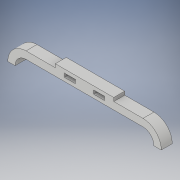
# Autodesk Inventor part: RadioPanelMountB
Saved by Autodesk Inventor 2018 (Build 220112000, 112)
## iProperties
Created: 2017-09-08
Part Number: RadioPanelMountB
Material: Generic
Document SubType Name: Modeling
Designer: Srinity
Density: 1 g/cm^3
Appearance: Default
Author: Srinity
Autodesk Inventor part; units mm, degrees
ref_plane "YZ Plane" through (0, 0, 0) normal (1, 0, 0) x (0, 1, 0)
ref_plane "XZ Plane" through (0, 0, 0) normal (0, 1, 0) x (-1, 0, 0)
ref_plane "XY Plane" through (0, 0, 0) normal (0, 0, 1) x (1, 0, 0)
sketch "Sketch1" plane through (0, 0, 0) normal (0, 0, 1) x (1, 0, 0)
  line L0 (-25.4, 9.398) -> (25.4, 9.398)
  line L1 (25.4, 9.398) -> (25.4, 6.35)
  line L2 (-25.4, 6.35) -> (-25.4, 9.398)
  line L3 (-50.8, 6.35) -> (-25.4, 6.35)
  line L4 (50.8, 6.35) -> (50.8, 0) construction
  line L5 (50.8, 0) -> (-50.8, 0)
  line L6 (-50.8, 0) -> (-50.8, 6.35) construction
  arc A0 (-50.8, 6.35) -> (-66.675, -9.525) centre (-50.8, -9.525) ccw
  arc A1 (38.1, 0) -> (66.675, -9.525) centre (50.8, -9.525) ccw construction
  arc A2 (-60.325, -9.525) -> (-50.8, -19.05) centre (-50.8, -9.525) ccw construction
  arc A3 (50.8, 0) -> (60.325, -9.525) centre (50.8, -9.525) ccw construction
  line L7 (25.4, 6.35) -> (50.8, 6.35)
  line L8 (-60.325, -9.525) -> (-66.675, -9.525)
  arc A4 (-50.8, 0) -> (-60.325, -9.525) centre (-50.8, -9.525) ccw
  arc A5 (60.325, -9.525) -> (50.8, 0) centre (50.8, -9.525) ccw
  arc A6 (-38.1, 0) -> (-50.8, 6.35) centre (-50.8, -9.525) ccw construction
  arc A7 (50.8, 6.35) -> (38.1, 0) centre (50.8, -9.525) ccw construction
  arc A8 (66.675, -9.525) -> (50.8, 6.35) centre (50.8, -9.525) ccw
  arc A9 (-66.675, -9.525) -> (-38.1, 0) centre (-50.8, -9.525) ccw construction
  arc A10 (-50.8, -19.05) -> (-50.8, 0) centre (-50.8, -9.525) ccw construction
  line L9 (66.675, -9.525) -> (60.325, -9.525)
  point P0 (0, 0)
  point P1 (50.8, 3.175)
  point P2 (-50.8, 3.175)
  dimension "d0" = 50.8
  dimension "d1" = 3.048
  dimension "d2" = 6.35
  dimension "d3" = 25.4
  dimension "d4" = 25.4
  dimension "d5" = 25.4
  dimension "d8" = 9.525
  constraints: 22 point on circle, 20 end point, 11 centre point, 6 tangent, 4 horizontal, 4 parallel, 4 point on line, 3 midpoint, 3 perpendicular, 2 coincident, 2 collinear, 2 equal radius, 2 vertical alignment
  measures "d0" distance of L0.start L0.end
  measures "d1" distance of L0.end L1.end
  measures "d2" distance between parallel lines of L5 L3
  measures "d3" distance of L3.start L2.start
  measures "d4" distance of L1.end L4.start
  measures "d5" distance from line of L2 point (0, 0)
  measures "d8" radius of A4
extrude "Extrusion1" add sketch "Sketch1" along normal blind 9.525
sketch "Sketch2" plane through (0, 0, 9.525) normal (0, 0, 1) x (1, 0, 0)
  line L0 (17.4625, 3.175) -> (7.9375, 3.175)
  line L1 (7.9375, 3.175) -> (7.9375, 6.35)
  line L2 (7.9375, 6.35) -> (17.4625, 6.35)
  line L3 (17.4625, 6.35) -> (17.4625, 3.175)
  line L4 (-7.9375, 3.175) -> (-17.4625, 3.175)
  line L5 (-17.4625, 3.175) -> (-17.4625, 6.35)
  line L6 (-17.4625, 6.35) -> (-7.9375, 6.35)
  line L7 (-7.9375, 6.35) -> (-7.9375, 3.175)
  line L8 (12.7, 3.175) -> (12.7, 6.35) construction
  line L9 (-12.7, 3.175) -> (-12.7, 6.35) construction
  line L10 (-50.8, 0) -> (50.8, 0) projected
  point P0 (0, 0)
  dimension "d11" = 9.525
  dimension "d12" = 3.175
  dimension "d13" = 12.7
  dimension "d14" = 12.7
  dimension "d15" = 3.175
  constraints: 20 end point, 4 midpoint, 4 parallel, 3 collinear, 2 horizontal, 2 perpendicular
  measures "d11" distance of L0.start L0.end
  measures "d12" distance of L0.end L1.end
  measures "d13" distance from line of L8 point (0, 0)
  measures "d14" distance from line of point (0, 0) L9
  measures "d15" distance between parallel lines of L10 L0
extrude "Extrusion2" cut sketch "Sketch2" against normal through all
equation "\"d5\" = 0.5 * d0"
body "Solid1"
